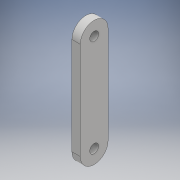
# Autodesk Inventor part: korba
Saved by Autodesk Inventor 2017 (Build 210142000, 142)
## iProperties
Created: 2017-05-09
Part Number: korba
Material: Ogólny
Document SubType Name: Modeling
Designer: Damian
Density: 1 g/cm^3
Appearance: Domyślna
Author: Damian
Autodesk Inventor part; units mm, degrees
ref_plane "YZ Plane" through (0, 0, 0) normal (1, 0, 0) x (0, 1, 0)
ref_plane "XZ Plane" through (0, 0, 0) normal (0, 1, 0) x (-1, 0, 0)
ref_plane "XY Plane" through (0, 0, 0) normal (0, 0, 1) x (1, 0, 0)
sketch "Szkic1" plane through (0, 0, 0) normal (1, 0, 0) x (0, 1, 0)
  line L0 (5, 0) -> (5, 0)
  line L1 (10, 5) -> (10, 40)
  line L2 (5, 45) -> (5, 45)
  line L3 (0, 40) -> (0, 5)
  arc A0 (10, 40) -> (5, 45) centre (5, 40) ccw
  arc A1 (5, 45) -> (0, 40) centre (5, 40) ccw
  arc A2 (5, 0) -> (10, 5) centre (5, 5) ccw
  arc A3 (0, 5) -> (5, 0) centre (5, 5) ccw
  circle A4 centre (5, 40) radius 1.6
  circle A5 centre (5, 5) radius 1.6
  point P0 (0, 0)
  point P1 (10, 45)
  point P2 (0, 45)
  dimension "d0" = 10
  dimension "d2" = 5
  dimension "d3" = 35
  dimension "d4" = 3.2
  dimension "d5" = 3.2
  constraints: 8 end point, 8 point on circle, 8 tangent, 6 centre point, 6 point on line, 3 equal radius, 2 coincident, 2 parallel, 1 horizontal, 1 perpendicular
  measures "d0" distance of point (0, 45) point (10, 45)
  measures "d2" radius of A0
  measures "d3" distance of A2.centre A0.centre
  measures "d4" diameter of A4
  measures "d5" diameter of A5
extrude "Wyciągnięcie proste1" add sketch "Szkic1" along normal blind 3
